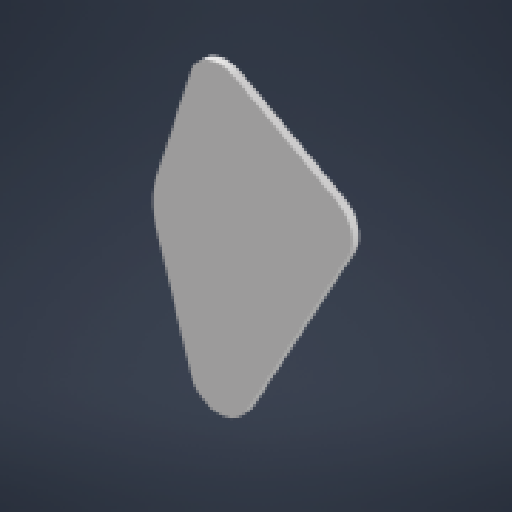
# Autodesk Inventor part: pto-linear-guide
Saved by Autodesk Inventor 2023.2 (Build 272271000, 271)
## iProperties
Created: 2023-03-20
Part Number: pto-linear-guide
Material: Generic
Document SubType Name: Modeling
Designer: Liam
Density: 1 g/cm^3
Appearance: Default
Author: Liam
Autodesk Inventor part; units mm, degrees
ref_plane "YZ Plane" through (0, 0, 0) normal (1, 0, 0) x (0, 1, 0)
ref_plane "XZ Plane" through (0, 0, 0) normal (0, 1, 0) x (-1, 0, 0)
ref_plane "XY Plane" through (0, 0, 0) normal (0, 0, 1) x (1, 0, 0)
sketch "Sketch1" plane through (0, 0, 0) normal (0, 0, 1) x (1, 0, 0)
  circle A0 centre (0, 38.1) radius 2.1844 projected
  circle A1 centre (0, 25.4) radius 2.1844 projected
  circle A2 centre (0, 76.2) radius 2.1844 projected
  circle A3 centre (0, 63.5) radius 2.1844 projected
  line L0 (23.4735, 61.2055) -> (19.7174, 61.053)
  line L1 (17.7073, 64.2296) -> (19.7174, 61.053)
  line L2 (17.7073, 64.2296) -> (19.4532, 67.5588)
  line L3 (23.2093, 67.7113) -> (19.4532, 67.5588)
  line L4 (23.2093, 67.7113) -> (25.2195, 64.5347)
  line L5 (25.2195, 64.5347) -> (23.4735, 61.2055)
  circle A4 centre (0, 50.8) radius 7.62
  line L6 (27.0259, 61.3194) -> (5.5626, 22.3373)
  line L7 (24.5261, 69.9447) -> (3.0628, 81.7625)
  line L8 (-6.0575, 78.105) -> (-13.3265, 54.991)
  line L9 (-6.0575, 23.495) -> (-13.3265, 46.609)
  arc A5 (-6.0575, 23.495) -> (5.5626, 22.3373) centre (0, 25.4) ccw
  arc A6 (3.0628, 81.7625) -> (-6.0575, 78.105) centre (0, 76.2) ccw
  arc A7 (27.0259, 61.3194) -> (24.5261, 69.9447) centre (21.4634, 64.3821) ccw
  arc A8 (-13.3265, 54.991) -> (-13.3265, 46.609) centre (0, 50.8) ccw
  point P0 (0, 0)
  point P1 (23.4238, 61.2841)
  point P2 (10.7317, 70.2911)
  dimension "d10" = 15.24
  constraints: 20 end point, 8 point on circle, 5 centre point, 3 parallel, 1 coincident, 8 other
  measures "d10" diameter of A4
extrude "Extrusion1" add sketch "Sketch1" along normal blind 1.524 contours A0 | A1 | A2 | A3 | L0 L1 L2 L3 L4 L5 | A4 | L6 A5 L9 A8 L8 A6 L7 A7
body "Solid1"
